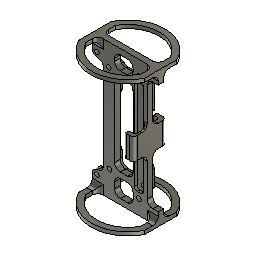
RISE_SensorMount (Autodesk Fusion 360 design; units mm, degrees)
Autodesk Fusion 360 part; units mm, degrees
(part 1 of 2)
sketch "Sketch1" plane through (0, 0, 0) normal (0, 0, 1) x (1, 0, 0)
  circle A0 centre (0, 0) radius 20
  line L0 (15, -5) -> (-15, -5)
  line L1 (-15, -5) -> (-15, 5)
  line L2 (-15, 5) -> (15, 5)
  line L3 (15, 5) -> (15, -5)
  line L4 (15, -5) -> (-15, 5) construction
  line L5 (-15, -5) -> (15, 5) construction
  dimension "d1" = 40
  dimension "d2" = 30
  dimension "d3" = 10
  constraint coincident A0.centre origin
  constraint horizontal L0
  constraint perpendicular L0 L1
  constraint parallel L0 L2
  constraint parallel L1 L3
  constraint coincident L4 A0.centre
  constraint coincident L5 A0.centre
  measures "d1" diameter of A0
  measures "d2" distance of L1.end L2.end
  measures "d3" distance of L0.end L1.end
extrude "Extrude1" add sketch "Sketch1" along normal blind 70 contours L0 L1 L2 L3 makes body 1
extrude "Extrude2" add sketch "Sketch1" against normal blind 3 separate body makes body 2
extrude "Extrude3" add sketch "Sketch1" against normal blind 3 contours L0 L1 L2 L3 bodies 1 2
sketch "Sketch2" plane through (0, 0, 70) normal (0, 0, 1) x (-1, 0, 0)
  line L0 (-15, -5) -> (15, -5)
  line L1 (15, -5) -> (15, 5)
  line L2 (15, 5) -> (-15, 5)
  line L3 (-15, 5) -> (-15, -5)
  circle A0 centre (0, 0) radius 20
  constraint coincident A0.centre origin
extrude "Extrude4" add sketch "Sketch2" along normal blind 3 contours L0 L1 L2 L3 | A0 bodies 1
sketch "Sketch3" plane through (0, -5, 0) normal (0, -1, 0) x (1, 0, 0)
  line L0 (-15, 0) -> (15, 0)
  line L1 (15, 0) -> (15, 70)
  line L2 (15, 70) -> (-15, 70)
  line L3 (-15, 70) -> (-15, 0)
  circle A0 centre (-11.5, 64) radius 1.25
  circle A1 centre (11.5, 64) radius 1.25
  circle A2 centre (-11.5, 6) radius 1.25
  circle A3 centre (11.5, 6) radius 1.25
  line L4 (-14, 59.5) -> (-14, 10.5)
  line L5 (-9, 10.5) -> (-9, 59.5)
  line L6 (9, 10.5) -> (9, 59.5)
  line L7 (14, 59.5) -> (14, 10.5)
  line L8 (10.5, 9) -> (12.5, 9)
  line L9 (10.5, 61) -> (12.5, 61)
  line L10 (-12.5, 61) -> (-10.5, 61)
  line L11 (-12.5, 9) -> (-10.5, 9)
  arc A4 (-12.5, 61) -> (-14, 59.5) centre (-12.5, 59.5) ccw
  arc A5 (-9, 59.5) -> (-10.5, 61) centre (-10.5, 59.5) ccw
  arc A6 (-14, 10.5) -> (-12.5, 9) centre (-12.5, 10.5) ccw
  arc A7 (-10.5, 9) -> (-9, 10.5) centre (-10.5, 10.5) ccw
  arc A8 (9, 10.5) -> (10.5, 9) centre (10.5, 10.5) ccw
  arc A9 (12.5, 9) -> (14, 10.5) centre (12.5, 10.5) ccw
  arc A10 (14, 59.5) -> (12.5, 61) centre (12.5, 59.5) ccw
  arc A11 (10.5, 61) -> (9, 59.5) centre (10.5, 59.5) ccw
  dimension "d13" = 23
  dimension "d14" = 58
  dimension "d15" = 2.5
  dimension "d16" = 2.5
  dimension "d17" = 2.5
  dimension "d18" = 2.5
  dimension "d20" = 1.5
  dimension "d21" = 1.5
  dimension "d22" = 1.5
  dimension "d23" = 1.5
  dimension "d24" = 1.5
  dimension "d25" = 1.5
  dimension "d26" = 1.5
  dimension "d27" = 1.5
  constraint perpendicular L7 L8
  constraint perpendicular L7 L9
  constraint perpendicular L5 L10
  constraint perpendicular L5 L11
  constraint tangent L4 A4
  constraint tangent L10 A4
  constraint tangent L5 A5
  constraint tangent L10 A5
  constraint tangent L4 A6
  constraint tangent L11 A6
  constraint tangent L5 A7
  constraint tangent L11 A7
  constraint tangent L6 A8
  constraint tangent L8 A8
  constraint tangent L8 A9
  constraint tangent L7 A9
  constraint tangent L7 A10
  constraint tangent L9 A10
  constraint tangent L6 A11
  constraint tangent L9 A11
  measures "d13" distance of A0.centre A1.centre
  measures "d14" distance of A0.centre A2.centre
  measures "d15" diameter of A0
  measures "d16" diameter of A1
  measures "d17" diameter of A2
  measures "d18" diameter of A3
  measures "d20" radius of A4
  measures "d21" radius of A5
  measures "d22" radius of A6
  measures "d23" radius of A7
  measures "d24" radius of A8
  measures "d25" radius of A9
  measures "d26" radius of A10
  measures "d27" radius of A11
extrude "Extrude5" cut sketch "Sketch3" against normal blind 2 contours L4 L5 L10 L11 A4 A5 A6 A7 | L6 L7 L8 L9 A8 A9 A10 A11 bodies 1
extrude "Extrude6" cut 1 faces at (3, -5, 26.8333) along direction (0, 1, 0) blind 2.5 on bodies 1 bodies 1
extrude "Extrude7" cut 2 faces at (-10.6667, -3, 26.8333) (12.3333, -3, 43.1667) along direction (0, 1, 0) blind 2.5 on bodies 1 bodies 1
extrude "Extrude8" cut 1 faces at (-5, 5, 23.3333) along direction (0, -1, 0) blind 2.5 on bodies 1 bodies 1
extrude "Extrude9" cut sketch "Sketch3" against normal blind 100 contours A2 | A3 bodies 1
extrude "Extrude10" cut sketch "Sketch3" against normal blind 100 contours A0 | A1 bodies 1
sketch "Sketch4" plane through (0, 2.5, 0) normal (0, 1, 0) x (-1, 0, 0)
  circle A0 centre (11.5, 64) radius 1.25
  circle A1 centre (-11.5, 64) radius 1.25
  circle A2 centre (11.5, 6) radius 1.25
  circle A3 centre (-11.5, 6) radius 1.25
  line L0 (-15, 0) -> (15, 0)
  line L1 (15, 0) -> (15, 70)
  line L2 (15, 70) -> (-15, 70)
  line L3 (-15, 70) -> (-15, 0)
  line L4 (0, 0) -> (0, 9)
  line L5 (0, 9) -> (0, 12)
  line L6 (0, 12) -> (7.25, 12)
  line L7 (0, 12) -> (-7.25, 12)
  circle A4 centre (-8.5, 12) radius 1.25
  circle A5 centre (8.5, 12) radius 1.25
  line L8 (0, 12) -> (0, 21.5)
  line L9 (0, 0) -> (0, 21.5)
  line L10 (0, 24.5) -> (0, 35)
  line L11 (0, 70) -> (0, 60)
  line L12 (0, 60) -> (9, 60)
  line L13 (0, 60) -> (-9, 60)
  line L14 (0, 60) -> (0, 45)
  line L15 (9.5, 43.5) -> (-9.5, 43.5)
  line L16 (-10.5, 44.5) -> (-10.5, 45.5)
  line L17 (-9.5, 46.5) -> (9.5, 46.5)
  line L18 (10.5, 45.5) -> (10.5, 44.5)
  line L19 (10.5, 43.5) -> (-10.5, 46.5) construction
  line L20 (-10.5, 43.5) -> (10.5, 46.5) construction
  line L21 (0, 35) -> (0, 45)
  line L22 (0, 21.5) -> (0, 23)
  line L23 (8.5, 24.5) -> (-8.5, 24.5)
  line L24 (-9.5, 23.5) -> (-9.5, 22.5)
  line L25 (-8.5, 21.5) -> (8.5, 21.5)
  line L26 (9.5, 22.5) -> (9.5, 23.5)
  line L27 (9.5, 24.5) -> (-9.5, 21.5) construction
  line L28 (-9.5, 24.5) -> (9.5, 21.5) construction
  circle A6 centre (-9, 60) radius 1.25
  circle A7 centre (9, 60) radius 1.25
  arc A8 (-9.5, 46.5) -> (-10.5, 45.5) centre (-9.5, 45.5) ccw
  arc A9 (-10.5, 44.5) -> (-9.5, 43.5) centre (-9.5, 44.5) ccw
  arc A10 (10.5, 45.5) -> (9.5, 46.5) centre (9.5, 45.5) ccw
  arc A11 (9.5, 43.5) -> (10.5, 44.5) centre (9.5, 44.5) ccw
  arc A12 (-9.5, 22.5) -> (-8.5, 21.5) centre (-8.5, 22.5) ccw
  arc A13 (-8.5, 24.5) -> (-9.5, 23.5) centre (-8.5, 23.5) ccw
  arc A14 (9.5, 23.5) -> (8.5, 24.5) centre (8.5, 23.5) ccw
  arc A15 (8.5, 21.5) -> (9.5, 22.5) centre (8.5, 22.5) ccw
  point P0 (0, 45)
  point P1 (0, 23)
  dimension "d40" = 9
  dimension "d48" = 3
  dimension "d49" = 8.5
  dimension "d50" = 8.5
  dimension "d51" = 2.5
  dimension "d52" = 2.5
  dimension "d74" = 35
  dimension "d75" = 10
  dimension "d76" = 9
  dimension "d77" = 9
  dimension "d78" = 15
  dimension "d79" = 21
  dimension "d80" = 3
  dimension "d81" = 19
  dimension "d82" = 3
  dimension "d83" = 2.5
  dimension "d84" = 2.5
  dimension "d85" = 1
  dimension "d86" = 1
  dimension "d87" = 1
  dimension "d88" = 1
  dimension "d89" = 1
  dimension "d90" = 1
  dimension "d91" = 1
  dimension "d92" = 1
  constraint coincident L4.start L9.start
  constraint perpendicular L0 L4
  constraint parallel L4 L5
  constraint perpendicular L5 L6
  constraint perpendicular L5 L7
  constraint coincident A5 L6.end
  constraint coincident A4 L7.end
  constraint collinear L9 L10
  constraint midpoint L2 L11.start
  constraint perpendicular L2 L11
  constraint perpendicular L11 L12
  constraint perpendicular L11 L13
  constraint perpendicular L12 L14
  constraint horizontal L15
  constraint perpendicular L15 L16
  constraint parallel L15 L17
  constraint parallel L16 L18
  constraint coincident L19 P0
  constraint coincident L20 P0
  constraint coincident P0 L14.end
  constraint parallel L8 L22
  constraint horizontal L23
  constraint perpendicular L23 L24
  constraint parallel L23 L25
  constraint parallel L24 L26
  constraint coincident L27 P1
  constraint coincident L28 P1
  constraint coincident P1 L22.end
  constraint coincident L13.end A6.centre
  constraint coincident L12.end A7.centre
  constraint coincident L19.end L16
  constraint coincident L19.end L17
  constraint tangent L16 A8
  constraint tangent L17 A8
  constraint coincident L20.start L16
  constraint coincident L20.start L15
  constraint tangent L16 A9
  constraint tangent L15 A9
  constraint coincident L20.end L17
  constraint coincident L20.end L18
  constraint tangent L17 A10
  constraint tangent L18 A10
  constraint coincident L19.start L15
  constraint coincident L19.start L18
  constraint tangent L15 A11
  constraint tangent L18 A11
  constraint coincident L27.end L25
  constraint coincident L27.end L24
  constraint tangent L25 A12
  constraint tangent L24 A12
  constraint coincident L28.start L24
  constraint coincident L28.start L23
  constraint tangent L24 A13
  constraint tangent L23 A13
  constraint coincident L27.start L23
  constraint coincident L27.start L26
  constraint tangent L23 A14
  constraint tangent L26 A14
  constraint coincident L28.end L25
  constraint coincident L28.end L26
  constraint tangent L25 A15
  constraint tangent L26 A15
  measures "d40" distance of L4.start L4.end
  measures "d48" distance of L4.end L5.end
  measures "d49" distance of L5.end A5.centre
  measures "d50" distance of L5.end A4.centre
  measures "d51" diameter of A4
  measures "d52" diameter of A5
  measures "d74" distance of L4.start L10.end
  measures "d75" distance of L11.start L11.end
  measures "d76" distance of L11.end L12.end
  measures "d77" distance of L11.end L13.end
  measures "d78" distance of L11.end P0
  measures "d79" distance of L19.end L20.end
  measures "d80" distance of L20.start L19.end
  measures "d81" distance of L27.end L28.end
  measures "d82" distance of L28.start L27.end
  measures "d83" diameter of A6
  measures "d84" diameter of A7
  measures "d85" radius of A8
  measures "d86" radius of A9
  measures "d87" radius of A10
  measures "d88" radius of A11
  measures "d89" radius of A12
  measures "d90" radius of A13
  measures "d91" radius of A14
  measures "d92" radius of A15
extrude "Extrude15" cut sketch "Sketch4" against normal blind 100 contours A6 bodies 1
extrude "Extrude16" cut sketch "Sketch4" against normal blind 100 contours A4 | A5 | A7 bodies 1
extrude "Extrude17" cut sketch "Sketch4" against normal blind 2 contours L23 L24 L25 L26 A12 A13 A14 A15 | L14 L15 L17 L18 L21 A10 A11 | L14 L15 L16 L17 L21 A8 A9 bodies 1
extrude "Extrude18" add 1 faces at (-15, -0.8333, 23.3333) along direction (-1, 0, 0) blind 3 on bodies 1 bodies 1
extrude "Extrude19" add 1 faces at (15, 0.8333, 23.3333) along direction (1, 0, 0) blind 3 on bodies 1 bodies 1
sketch "Sketch5" plane through (0, 0, 70) normal (0, 0, -1) x (1, 0, 0)
  line L0 (18, -2.5) -> (-18, -2.5)
  line L1 (-18, -2.5) -> (-18, 2.5)
  line L2 (-18, 2.5) -> (18, 2.5)
  line L3 (18, 2.5) -> (18, -2.5)
  circle A0 centre (0, 0) radius 20
  line L4 (18, -2.5) -> (18, -8.7178)
  line L5 (18, -8.7178) -> (18, 2.5)
  line L6 (18, 2.5) -> (18, 8.7178)
  line L7 (-18, 2.5) -> (-18, 8.7178)
  line L8 (-18, -2.5) -> (-18, -8.7178)
  constraint coincident L0.start L3.end
  constraint coincident A0 L4.end
  constraint perpendicular L0 L4
  constraint coincident L2.end L3.start
  constraint coincident A0 L6.end
  constraint perpendicular L2 L6
  constraint coincident L1.end L2.start
  constraint coincident A0 L7.end
  constraint perpendicular L2 L7
  constraint coincident L0.end L1.start
  constraint coincident A0 L8.end
  constraint perpendicular L0 L8
extrude "Extrude20" cut sketch "Sketch5" against normal blind 10 contours L3 A0 L4 L5 L6 | L1 A0 L7 L8 bodies 1
sketch "Sketch6" plane through (0, 0, 0) normal (0, 0, 1) x (-1, 0, 0)
  line L0 (-18, 2.5) -> (18, 2.5)
  line L1 (18, 2.5) -> (18, -2.5)
  line L2 (18, -2.5) -> (-18, -2.5)
  line L3 (-18, -2.5) -> (-18, 2.5)
  circle A0 centre (0, 0) radius 20
  line L4 (18, 2.5) -> (18, 8.7178)
  line L5 (18, 8.7178) -> (18, -8.7178)
  line L6 (-18, -2.5) -> (-18, -8.7178)
  line L7 (-18, -8.7178) -> (-18, 8.7178)
  constraint coincident L0.end L1.start
  constraint coincident A0 L4.end
  constraint perpendicular L0 L4
  constraint coincident A0 L5.end
  constraint perpendicular L2 L5
  constraint coincident L2.end L3.start
  constraint coincident A0 L6.end
  constraint perpendicular L2 L6
  constraint coincident A0 L7.end
  constraint perpendicular L0 L7
extrude "Extrude21" cut sketch "Sketch6" against normal blind 10 contours L3 A0 L6 L7 bodies 1
extrude "Extrude22" cut sketch "Sketch6" against normal blind 10 contours L1 A0 L4 L5 bodies 1
extrude "Extrude23" cut 2 faces at (-12.3867, -0.5, 27.6871) (12.3867, -0.5, 27.6871) along direction (0, 1, 0) blind 1 on bodies 1 bodies 1
extrude "Extrude24" cut 1 faces at (-2.7544, -2.5, 43.6171) along direction (0, 1, 0) blind 1 on bodies 1 bodies 1
extrude "Extrude25" cut 1 faces at (-2.8333, 2.5, 37.1667) along direction (0, -1, 0) blind 1 on bodies 1 bodies 1
extrude "Extrude26" cut 2 faces at (3, 0.5, 44.5) (-2.8333, 0.5, 22.5) along direction (0, -1, 0) blind 1 on bodies 1 bodies 1
extrude "Extrude27" cut 1 faces at (6.499, 3.7661, 73) along direction (0, 0, -1) blind 1 on bodies 1 bodies 1
extrude "Extrude28" cut 1 faces at (4.8796, -1.2694, -3) along direction (0, 0, 1) blind 1 on bodies 1 bodies 1
sketch "Sketch7" plane through (0, 0, -2) normal (0, 0, -1) x (1, 0, 0)
  line L0 (-18, 8.7178) -> (-18, -8.7178)
  arc A0 (-18, -8.7178) -> (18, -8.7178) centre (0, 0) ccw
  line L1 (18, -8.7178) -> (18, 8.7178)
  arc A1 (18, 8.7178) -> (-18, 8.7178) centre (0, 0) ccw
  circle A2 centre (0, 0) radius 17
  line L2 (-18, 0) -> (-15, 0)
  line L3 (-15, 0) -> (-15, 8)
  line L4 (-15, 0) -> (-15, -8)
  line L5 (18, 0) -> (15, 0)
  line L6 (15, 0) -> (15, -8)
  line L7 (15, 0) -> (15, 8)
  line L8 (0, 0) -> (0, 1.5)
  line L9 (0, 0) -> (0, -1.5)
  line L10 (0, -1.5) -> (15, -1.5)
  line L11 (0, -1.5) -> (-15, -1.5)
  line L12 (0, 1.5) -> (-15, 1.5)
  line L13 (0, 1.5) -> (15, 1.5)
  dimension "d131" = 34
  dimension "d132" = 1.5
  dimension "d133" = 1.5
  constraint concentric A0 A2
  constraint midpoint L0 L2.start
  constraint perpendicular L0 L2
  constraint coincident A2 L3.end
  constraint perpendicular L2 L3
  constraint coincident A2 L4.end
  constraint perpendicular L2 L4
  constraint midpoint L1 L5.start
  constraint perpendicular L1 L5
  constraint coincident A2 L6.end
  constraint perpendicular L5 L6
  constraint coincident A2 L7.end
  constraint perpendicular L5 L7
  constraint coincident A0.centre A1.centre
  constraint parallel L6 L8
  constraint parallel L8 L9
  constraint coincident L6 L10.end
  constraint perpendicular L6 L10
  constraint coincident L4 L11.end
  constraint perpendicular L4 L11
  constraint perpendicular L8 L12
  constraint coincident L7 L13.end
  constraint perpendicular L7 L13
  measures "d131" diameter of A2
  measures "d132" distance of A0.centre L8.end
  measures "d133" distance of A0.centre L9.end
extrude "Extrude29" cut sketch "Sketch7" against normal blind 100 contours A2 L3 L7 L12 L13 | A2 L4 L6 L10 L11 bodies 1
sketch "Sketch8" plane through (0, -1.5, 0) normal (0, -1, 0) x (1, 0, 0)
  arc A0 (-9, 58.75) -> (-9.895, 60.8726) centre (-9, 60) ccw
  line L0 (-9, 58.75) -> (-9, 13.1456)
  arc A1 (-9, 10.8544) -> (-9, 13.1456) centre (-8.5, 12) ccw
  line L1 (-9, 10.8544) -> (-9, 10.5)
  arc A2 (-10.5, 9) -> (-9, 10.5) centre (-10.5, 10.5) ccw
  line L2 (-10.5, 9) -> (-12.5, 9)
  arc A3 (-14, 10.5) -> (-12.5, 9) centre (-12.5, 10.5) ccw
  line L3 (-14, 10.5) -> (-14, 59.5)
  arc A4 (-12.5, 61) -> (-14, 59.5) centre (-12.5, 59.5) ccw
  line L4 (-12.5, 61) -> (-10.5, 61)
  arc A5 (-9.895, 60.8726) -> (-10.5, 61) centre (-10.5, 59.5) ccw
  arc A6 (9, 13.1456) -> (9, 10.8544) centre (8.5, 12) ccw
  line L5 (9, 13.1456) -> (9, 58.75)
  arc A7 (9.895, 60.8726) -> (9, 58.75) centre (9, 60) ccw
  arc A8 (10.5, 61) -> (9.895, 60.8726) centre (10.5, 59.5) ccw
  line L6 (10.5, 61) -> (12.5, 61)
  arc A9 (14, 59.5) -> (12.5, 61) centre (12.5, 59.5) ccw
  line L7 (14, 59.5) -> (14, 10.5)
  arc A10 (12.5, 9) -> (14, 10.5) centre (12.5, 10.5) ccw
  line L8 (12.5, 9) -> (10.5, 9)
  arc A11 (9, 10.5) -> (10.5, 9) centre (10.5, 10.5) ccw
  line L9 (9, 10.5) -> (9, 10.8544)
  circle A12 centre (11.5, 6) radius 1.25
  circle A13 centre (-11.5, 6) radius 1.25
  circle A14 centre (11.5, 64) radius 1.25
  circle A15 centre (-11.5, 64) radius 1.25
  line L10 (15, 70) -> (15, 72)
  line L11 (15, 72) -> (-15, 72)
  line L12 (-15, 72) -> (-15, 70)
  line L13 (-18, 70) -> (-18, 0)
  line L14 (-15, 0) -> (-15, -2)
  line L15 (-15, -2) -> (15, -2)
  line L16 (15, -2) -> (15, 0)
  line L17 (18, 0) -> (18, 70)
  line L18 (0, -2) -> (-6, -2)
  line L19 (0, -2) -> (6, -2)
  line L20 (6, 7) -> (6, 63)
  line L21 (6, 72) -> (-6, 72)
  line L22 (-6, 63) -> (-6, 7)
  line L23 (6, -2) -> (6, 35)
  line L24 (6, 35) -> (0, 35)
  line L25 (6, -2) -> (6, 4)
  line L26 (-6, -2) -> (-6, 4)
  line L27 (6, 72) -> (6, 66)
  line L28 (3, 66) -> (-3, 66)
  line L29 (3, 4) -> (-3, 4)
  arc A16 (6, 63) -> (3, 66) centre (3, 63) ccw
  arc A17 (-3, 66) -> (-6, 63) centre (-3, 63) ccw
  arc A18 (3, 4) -> (6, 7) centre (3, 7) ccw
  arc A19 (-6, 7) -> (-3, 4) centre (-3, 7) ccw
  line L30 (15, 0) -> (18, 0)
  line L31 (18, 70) -> (15, 70)
  line L32 (-15, 70) -> (-18, 70)
  line L33 (-18, 0) -> (-15, 0)
  dimension "d138" = 6
  dimension "d139" = 6
  dimension "d140" = 12
  dimension "d141" = 6
  dimension "d142" = 6
  dimension "d143" = 6
  dimension "d144" = 3
  dimension "d145" = 3
  dimension "d146" = 3
  dimension "d147" = 3
  constraint midpoint L15 L18.start
  constraint perpendicular L0 L18
  constraint perpendicular L5 L19
  constraint coincident L11 L21.start
  constraint perpendicular L11 L20
  constraint perpendicular L20 L21
  constraint perpendicular L20 L24
  constraint perpendicular L15 L25
  constraint perpendicular L15 L26
  constraint perpendicular L11 L27
  constraint perpendicular L22 L28
  constraint coincident L20 L23.end
  constraint coincident L21.start L20
  constraint coincident L27.end L28
  constraint tangent L20 A16
  constraint tangent L28 A16
  constraint coincident L21.end L22
  constraint tangent L28 A17
  constraint tangent L22 A17
  constraint coincident L19.end L20
  constraint coincident L25.end L29
  constraint tangent L20 A18
  constraint tangent L29 A18
  constraint coincident L26.end L29
  constraint coincident L18.end L22
  constraint tangent L29 A19
  constraint tangent L22 A19
  measures "d138" distance of L18.start L18.end
  measures "d139" distance of L18.start L19.end
  measures "d140" distance of L21.start L21.end
  measures "d141" distance of L19.end L25.end
  measures "d142" distance of L18.end L26.end
  measures "d143" distance of L21.start L27.end
  measures "d144" radius of A16
  measures "d145" radius of A17
  measures "d146" radius of A18
  measures "d147" radius of A19
move_body "Move1" bodies 1 to x (1, 0, 0) y (0, 1, 0) z (0, 0, 1) at (3, 0, 0)
extrude "Extrude31" add 2 faces at (-8.1449, 0.5, 54.9242) (14.1491, 0.5, 54.9261) along direction (0, -1, 0) blind 2 on bodies 1 bodies 1
sketch "Sketch9" plane through (0, -1.5, 0) normal (0, -1, 0) x (1, 0, 0)
  circle A0 centre (12, 60) radius 1.25
  line L0 (12, 46.5) -> (12.5, 46.5)
  arc A1 (13.5, 45.5) -> (12.5, 46.5) centre (12.5, 45.5) ccw
  line L1 (13.5, 45.5) -> (13.5, 44.5)
  arc A2 (12.5, 43.5) -> (13.5, 44.5) centre (12.5, 44.5) ccw
  line L2 (12.5, 43.5) -> (12, 43.5)
  line L3 (12, 43.5) -> (12, 46.5)
  circle A3 centre (11.5, 12) radius 1.25
  circle A4 centre (-5.5, 12) radius 1.25
  arc A5 (-6.5, 22.5) -> (-6, 21.634) centre (-5.5, 22.5) ccw
  line L4 (-6.5, 22.5) -> (-6.5, 23.5)
  arc A6 (-6, 24.366) -> (-6.5, 23.5) centre (-5.5, 23.5) ccw
  line L5 (-6, 24.366) -> (-6, 21.634)
  circle A7 centre (-6, 60) radius 1.25
  line L6 (-6, 43.5) -> (-6.5, 43.5)
  arc A8 (-7.5, 44.5) -> (-6.5, 43.5) centre (-6.5, 44.5) ccw
  line L7 (-7.5, 44.5) -> (-7.5, 45.5)
  arc A9 (-6.5, 46.5) -> (-7.5, 45.5) centre (-6.5, 45.5) ccw
  line L8 (-6.5, 46.5) -> (-6, 46.5)
  line L9 (-6, 46.5) -> (-6, 43.5)
  arc A10 (12.5, 23.5) -> (12, 24.366) centre (11.5, 23.5) ccw
  line L10 (12.5, 23.5) -> (12.5, 22.5)
  arc A11 (12, 21.634) -> (12.5, 22.5) centre (11.5, 22.5) ccw
  line L11 (12, 21.634) -> (12, 24.366)
  circle A12 centre (14.5, 6) radius 1.25
  circle A13 centre (-8.5, 6) radius 1.25
  circle A14 centre (14.5, 64) radius 1.25
  circle A15 centre (-8.5, 64) radius 1.25
  line L12 (18, 70) -> (18, 72)
  line L13 (18, 72) -> (-12, 72)
  line L14 (-12, 72) -> (-12, 70)
  line L15 (-15, 70) -> (-15, 0)
  line L16 (-12, 0) -> (-12, -2)
  line L17 (-12, -2) -> (18, -2)
  line L18 (18, -2) -> (18, 0)
  line L19 (21, 0) -> (21, 70)
  line L20 (-10, 66) -> (16, 66)
  line L21 (16, 66) -> (16, 4)
  line L22 (16, 4) -> (-10, 4)
  line L23 (-10, 4) -> (-10, 66)
  line L24 (18, 0) -> (21, 0)
  line L25 (21, 70) -> (18, 70)
  line L26 (-12, 70) -> (-15, 70)
  line L27 (-15, 0) -> (-12, 0)
  constraint horizontal L20
  constraint vertical L21
  constraint horizontal L22
  constraint vertical L23
extrude "Extrude32" add sketch "Sketch9" against normal blind 1 contours L0 A1 L1 A2 L2 L3 | A5 L4 A6 L5 | L6 A8 L7 A9 L8 L9 | A10 L10 A11 L11 bodies 1
extrude "Extrude33" add sketch "Sketch9" against normal blind 3 contours A12 | A13 | A14 | A15 bodies 1
extrude "Extrude34" cut sketch "Sketch3" against normal blind 5 contours L4 L5 L10 L11 A4 A5 A6 A7 | L6 L7 L8 L9 A8 A9 A10 A11 bodies 1
move_body "Move2" bodies 1 to x (1, 0, 0) y (0, 1, 0) z (0, 0, 1) at (1, 0, 0)
extrude "Extrude35" cut sketch "Sketch3" against normal blind 100 contours A0 | A1 | A2 | A3 bodies 1
extrude "Extrude36" add 1 faces at (12, 0, 37.1667) along direction (0, -1, 0) blind 1.5 on bodies 1 bodies 1
extrude "Extrude37" cut sketch "Sketch3" against normal blind 5 contours L6 L7 L8 L9 A8 A9 A10 A11 bodies 1
extrude "Extrude38" add 1 faces at (-9.6667, 0, 26.8333) along direction (0, -1, 0) blind 2 on bodies 1 bodies 1
extrude "Extrude39" cut 1 faces at (-9.6667, -2, 26.8333) along direction (0, 1, 0) blind 0.5 on bodies 1 bodies 1
extrude "Extrude40" add 2 faces at (11.7309, 0, 50.5961) (11.6667, 0, 37.1667) along direction (0, -1, 0) blind 0.5 on bodies 1 bodies 1
sketch "Sketch10" plane through (22, 0, 0) normal (1, 0, 0) x (0, 1, 0)
  line L0 (-8.7178, -2) -> (8.7178, -2)
  line L1 (8.7178, -2) -> (8.7178, 0)
  line L2 (8.7178, 0) -> (1.5, 0)
  line L3 (1.5, 0) -> (1.5, 70)
  line L4 (1.5, 70) -> (8.7178, 70)
  line L5 (8.7178, 70) -> (8.7178, 72)
  line L6 (8.7178, 72) -> (-8.7178, 72)
  line L7 (-8.7178, 72) -> (-8.7178, 70)
  line L8 (-8.7178, 70) -> (-1.5, 70)
  line L9 (-1.5, 70) -> (-1.5, 0)
  line L10 (-1.5, 0) -> (-8.7178, 0)
  line L11 (-8.7178, 0) -> (-8.7178, -2)
  line L12 (0, -2) -> (0, 5)
  line L13 (0, 72) -> (0, 65)
  line L14 (0, 5) -> (0, 65)
  line L15 (1.5, 65) -> (-1.5, 65)
  line L16 (-1.5, 65) -> (-1.5, 5)
  line L17 (-1.5, 5) -> (1.5, 5)
  line L18 (1.5, 5) -> (1.5, 65)
  line L19 (1.5, 65) -> (-1.5, 5) construction
  line L20 (-1.5, 65) -> (1.5, 5) construction
  point P0 (0, 35)
  dimension "d170" = 7
  dimension "d171" = 7
  dimension "d172" = 60
  constraint midpoint L0 L12.start
  constraint perpendicular L6 L12
  constraint midpoint L6 L13.start
  constraint perpendicular L6 L13
  constraint horizontal L15
  constraint perpendicular L15 L16
  constraint parallel L15 L17
  constraint parallel L16 L18
  constraint coincident L19 P0
  constraint coincident L20 P0
  constraint midpoint L14 P0
  measures "d170" distance of L12.start L12.end
  measures "d171" distance of L13.start L13.end
  measures "d172" distance of L15.end L16.end
extrude "Extrude41" cut sketch "Sketch10" against normal blind 7 contours L9 L14 L15 L16 L17 | L3 L14 L15 L17 L18 bodies 1
sketch "Sketch11" plane through (0, -1.5, 0) normal (0, -1, 0) x (1, 0, 0)
  line L0 (15, 65) -> (22, 65)
  line L1 (22, 65) -> (22, 70)
  line L2 (22, 70) -> (19, 70)
  line L3 (19, 70) -> (19, 72)
  line L4 (19, 72) -> (-11, 72)
  line L5 (-11, 72) -> (-11, 70)
  line L6 (-11, 70) -> (-14, 70)
  line L7 (-14, 70) -> (-14, 0)
  line L8 (-14, 0) -> (-11, 0)
  line L9 (-11, 0) -> (-11, -2)
  line L10 (-11, -2) -> (19, -2)
  line L11 (19, -2) -> (19, 0)
  line L12 (19, 0) -> (22, 0)
  line L13 (22, 0) -> (22, 5)
  line L14 (22, 5) -> (15, 5)
  line L15 (15, 5) -> (15, 65)
  line L16 (10.5, 61) -> (12.25, 61)
  arc A0 (14, 59.25) -> (12.25, 61) centre (13, 60) ccw
  line L17 (14, 59.25) -> (14, 46.366)
  arc A1 (14.5, 45.5) -> (14, 46.366) centre (13.5, 45.5) ccw
  line L18 (14.5, 45.5) -> (14.5, 44.5)
  arc A2 (14, 43.634) -> (14.5, 44.5) centre (13.5, 44.5) ccw
  line L19 (14, 43.634) -> (14, 10.5)
  arc A3 (12.5, 9) -> (14, 10.5) centre (12.5, 10.5) ccw
  line L20 (12.5, 9) -> (10.5, 9)
  arc A4 (9, 10.5) -> (10.5, 9) centre (10.5, 10.5) ccw
  arc A5 (10.5, 61) -> (9, 59.5) centre (10.5, 59.5) ccw
  circle A6 centre (-11.5, 6) radius 1.25
  circle A7 centre (11.5, 6) radius 1.25
  circle A8 centre (-11.5, 64) radius 1.25
  circle A9 centre (11.5, 64) radius 1.25
  circle A10 centre (-5, 60) radius 1.25
  circle A11 centre (-4.5, 12) radius 1.25
  line L21 (14, 43.634) -> (14, 46.366)
  line L22 (9, 10.5) -> (9, 59.5)
  constraint coincident A2.start L19.start
  constraint coincident L17.end A1.end
extrude "Extrude42" add sketch "Sketch11" against normal blind 3 contours A1 L18 A2 L21 bodies 1
sketch "Sketch13" plane through (15, 0, 0) normal (1, 0, 0) x (0, 1, 0)
  line L0 (-1.5, 65) -> (-1.5, 5)
  line L1 (1.5, 5) -> (1.5, 65)
  line L2 (0, 7) -> (0, 63)
  line L3 (9, 41) -> (-9, 41)
  line L4 (-9, 41) -> (-9, 29)
  line L5 (-9, 29) -> (9, 29)
  line L6 (9, 29) -> (9, 41)
  line L7 (9, 41) -> (-9, 29) construction
  line L8 (-9, 41) -> (9, 29) construction
  line L9 (1.5, 65) -> (-1.5, 65)
  line L10 (-1.5, 5) -> (1.5, 5)
  point P0 (0, 35)
  dimension "d192" = 18
  dimension "d193" = 12
  constraint horizontal L3
  constraint perpendicular L3 L4
  constraint parallel L3 L5
  constraint parallel L4 L6
  constraint coincident L7 P0
  constraint coincident L8 P0
  constraint midpoint L2 P0
  measures "d192" distance of L4.end L5.end
  measures "d193" distance of L3.end L4.end
extrude "Extrude45" add sketch "Sketch13" along normal blind 1 contours L0 L2 L3 L5 | L0 L3 L4 L5 | L1 L2 L3 L5 | L1 L3 L5 L6 bodies 1
sketch "Sketch14" plane through (-14, 0, 0) normal (-1, 0, 0) x (0, -1, 0)
  line L0 (-8.7178, -2) -> (8.7178, -2)
  line L1 (8.7178, -2) -> (8.7178, 0)
  line L2 (8.7178, 0) -> (1.5, 0)
  line L3 (1.5, 0) -> (1.5, 70)
  line L4 (1.5, 70) -> (8.7178, 70)
  line L5 (8.7178, 70) -> (8.7178, 72)
  line L6 (8.7178, 72) -> (-8.7178, 72)
  line L7 (-8.7178, 72) -> (-8.7178, 70)
  line L8 (-8.7178, 70) -> (-1.5, 70)
  line L9 (-1.5, 70) -> (-1.5, 0)
  line L10 (-1.5, 0) -> (-8.7178, 0)
  line L11 (-8.7178, 0) -> (-8.7178, -2)
  line L12 (0, -2) -> (0, 72)
  line L13 (1.5, 60) -> (-1.5, 60)
  line L14 (-1.5, 60) -> (-1.5, 10)
  line L15 (-1.5, 10) -> (1.5, 10)
  line L16 (1.5, 10) -> (1.5, 60)
  line L17 (1.5, 60) -> (-1.5, 10) construction
  line L18 (-1.5, 60) -> (1.5, 10) construction
  point P0 (0, 35)
  dimension "d196" = 50
  constraint midpoint L0 L12.start
  constraint midpoint L6 L12.end
  constraint horizontal L13
  constraint perpendicular L13 L14
  constraint parallel L13 L15
  constraint parallel L14 L16
  constraint coincident L17 P0
  constraint coincident L18 P0
  constraint midpoint L12 P0
  measures "d196" distance of L13.end L14.end
extrude "Extrude46" cut sketch "Sketch14" against normal blind 5 contours L9 L12 L13 L14 L15 | L3 L12 L13 L15 L16 bodies 1
extrude "Extrude47" cut 1 faces at (-9, -0.5, 26.6667) along direction (1, 0, 0) blind 1 on bodies 1 bodies 1
extrude "Extrude48" cut 1 faces at (-12, 0.5, 10) along direction (0, 0, -1) blind 1.5 on bodies 1 bodies 1
extrude "Extrude49" cut 1 faces at (-10, 0.5, 60) along direction (0, 0, 1) blind 1.5 on bodies 1 bodies 1
extrude "Extrude50" add 2 faces at (15, -0.5, 13) (15, -0.5, 57) along direction (1, 0, 0) blind 1 on bodies 1 bodies 1
extrude "Extrude52" add 2 faces at (4.1667, -0.5, 44.5) (4.5, -0.5, 22.5) along direction (0, 1, 0) blind 0.5 on bodies 1 bodies 1
sketch "Sketch15" plane through (9, 0, 0) normal (1, 0, 0) x (0, 1, 0)
  line L0 (-0.5, 24.5) -> (-0.5, 43.5)
  line L1 (-0.5, 43.5) -> (0, 43.5)
  line L2 (0, 43.5) -> (0, 46.5)
  line L3 (0, 46.5) -> (-0.5, 46.5)
  line L4 (-0.5, 46.5) -> (-0.5, 59.5)
  line L5 (-0.5, 59.5) -> (-1.5, 59.5)
  line L6 (-1.5, 59.5) -> (-1.5, 10.5)
  line L7 (-1.5, 10.5) -> (-0.5, 10.5)
  line L8 (-0.5, 10.5) -> (-0.5, 21.5)
  line L9 (-0.5, 21.5) -> (0, 21.5)
  line L10 (0, 21.5) -> (0, 24.5)
  line L11 (0, 24.5) -> (-0.5, 24.5)
  line L12 (-0.5, 21.5) -> (-0.5, 24.5)
  line L13 (-0.5, 46.5) -> (-0.5, 43.5)
  constraint coincident L8.end L9.start
  constraint coincident L0.start L11.end
  constraint coincident L3.end L4.start
  constraint coincident L0.end L1.start
extrude "Extrude53" add sketch "Sketch15" along normal blind 5 contours L1 L2 L3 L13 bodies 1
extrude "Extrude54" add sketch "Sketch15" along normal blind 5 contours L9 L10 L11 L12 bodies 1
sketch "Sketch16" plane through (0, 1.5, 0) normal (0, 1, 0) x (-1, 0, 0)
  line L0 (-15, 29) -> (-16, 29)
  line L1 (-16, 29) -> (-16, 5)
  line L2 (-16, 5) -> (-22, 5)
  line L3 (-22, 5) -> (-22, 0)
  line L4 (-22, 0) -> (-19, 0)
  line L5 (-19, 0) -> (-19, -2)
  line L6 (-19, -2) -> (11, -2)
  line L7 (11, -2) -> (11, 0)
  line L8 (11, 0) -> (14, 0)
  line L9 (14, 0) -> (14, 8.5)
  line L10 (14, 8.5) -> (8, 8.5)
  line L11 (8, 8.5) -> (8, 61.5)
  line L12 (8, 61.5) -> (14, 61.5)
  line L13 (14, 61.5) -> (14, 70)
  line L14 (14, 70) -> (11, 70)
  line L15 (11, 70) -> (11, 72)
  line L16 (11, 72) -> (-19, 72)
  line L17 (-19, 72) -> (-19, 70)
  line L18 (-19, 70) -> (-22, 70)
  line L19 (-22, 70) -> (-22, 65)
  line L20 (-22, 65) -> (-16, 65)
  line L21 (-16, 65) -> (-16, 41)
  line L22 (-16, 41) -> (-15, 41)
  line L23 (5.5, 23.5) -> (5.5, 22.5)
  arc A0 (4.5, 21.5) -> (5.5, 22.5) centre (4.5, 22.5) ccw
  line L24 (4.5, 21.5) -> (-12.5, 21.5)
  arc A1 (-13.5, 22.5) -> (-12.5, 21.5) centre (-12.5, 22.5) ccw
  line L25 (-13.5, 22.5) -> (-13.5, 23.5)
  arc A2 (-12.5, 24.5) -> (-13.5, 23.5) centre (-12.5, 23.5) ccw
  line L26 (-12.5, 24.5) -> (4.5, 24.5)
  arc A3 (5.5, 23.5) -> (4.5, 24.5) centre (4.5, 23.5) ccw
  line L27 (5.5, 43.5) -> (-13.5, 43.5)
  arc A4 (-14, 43.634) -> (-13.5, 43.5) centre (-13.5, 44.5) ccw
  line L28 (-14, 43.634) -> (-14, 46.366)
  arc A5 (-13.5, 46.5) -> (-14, 46.366) centre (-13.5, 45.5) ccw
  line L29 (-13.5, 46.5) -> (5.5, 46.5)
  arc A6 (6.5, 45.5) -> (5.5, 46.5) centre (5.5, 45.5) ccw
  line L30 (6.5, 45.5) -> (6.5, 44.5)
  arc A7 (5.5, 43.5) -> (6.5, 44.5) centre (5.5, 44.5) ccw
  circle A8 centre (5, 60) radius 1.25
  circle A9 centre (4.5, 12) radius 1.25
  circle A10 centre (-12.5, 12) radius 1.25
  circle A11 centre (-13, 60) radius 1.25
  circle A12 centre (-11.5, 64) radius 1.25
  circle A13 centre (11.5, 64) radius 1.25
  circle A14 centre (-11.5, 6) radius 1.25
  circle A15 centre (11.5, 6) radius 1.25
  line L31 (6.5, 45) -> (-14.5, 45)
  line L32 (-14.5, 45) -> (-14.5, 43.5)
  line L33 (-14.5, 45) -> (-14.5, 46.5)
  line L34 (-14.5, 46.5) -> (-13, 46.5)
  line L35 (-14.5, 43.5) -> (-13, 43.5)
  line L36 (-13, 43.5) -> (-13, 46.5)
  line L37 (-15, 41) -> (-15, 29)
  dimension "d219" = 21
  dimension "d220" = 1.5
  dimension "d221" = 1.5
  constraint midpoint L30 L31.start
  constraint perpendicular L28 L31
  constraint perpendicular L31 L32
  constraint perpendicular L31 L33
  constraint coincident L29 L34.end
  constraint perpendicular L28 L34
  constraint coincident L27 L35.end
  constraint perpendicular L28 L35
  constraint perpendicular L31 L36
  measures "d219" distance of L31.start L31.end
  measures "d220" distance of L31.end L32.end
  measures "d221" distance of L31.end L33.end
extrude "Extrude55" cut sketch "Sketch16" against normal blind 1.5 contours A4 L28 L31 L32 L35 | L28 A5 L31 L33 L34 bodies 1
fillet "Fillet12" radius 1 2 edges at (14.5, 0.75, 43.5) (14.5, 0.75, 46.5) on bodies 1
extrude "Extrude56" add 2 faces at (7.1667, 0, 44.5) (1.1667, 0, 23.5) along direction (0, 1, 0) blind 1.5 on bodies 1 bodies 1
extrude "Extrude57" cut 1 faces at (10.6667, -0.5, 37.878) along direction (0, 1, 0) blind 0.5 on bodies 1 bodies 1
sketch "Sketch17" plane through (0, 1.5, 0) normal (0, 1, 0) x (-1, 0, 0)
  circle A0 centre (11.5, 6) radius 1.25
  circle A1 centre (-11.5, 6) radius 1.25
  circle A2 centre (11.5, 64) radius 1.25
  circle A3 centre (-11.5, 64) radius 1.25
  circle A4 centre (-13, 60) radius 1.25
  circle A5 centre (-12.5, 12) radius 1.25
  circle A6 centre (4.5, 12) radius 1.25
  circle A7 centre (5, 60) radius 1.25
  line L0 (8, 61.5) -> (14, 61.5)
  line L1 (14, 61.5) -> (14, 70)
  line L2 (14, 70) -> (11, 70)
  line L3 (11, 70) -> (11, 72)
  line L4 (11, 72) -> (-19, 72)
  line L5 (-19, 72) -> (-19, 70)
  line L6 (-19, 70) -> (-22, 70)
  line L7 (-22, 70) -> (-22, 65)
  line L8 (-22, 65) -> (-16, 65)
  line L9 (-16, 65) -> (-16, 41)
  line L10 (-16, 41) -> (-15, 41)
  line L11 (-15, 41) -> (-15, 29)
  line L12 (-15, 29) -> (-16, 29)
  line L13 (-16, 29) -> (-16, 5)
  line L14 (-16, 5) -> (-22, 5)
  line L15 (-22, 5) -> (-22, 0)
  line L16 (-22, 0) -> (-19, 0)
  line L17 (-19, 0) -> (-19, -2)
  line L18 (-19, -2) -> (11, -2)
  line L19 (11, -2) -> (11, 0)
  line L20 (11, 0) -> (14, 0)
  line L21 (14, 0) -> (14, 8.5)
  line L22 (14, 8.5) -> (8, 8.5)
  line L23 (8, 8.5) -> (8, 61.5)
  line L24 (3.75, 60) -> (3.75, 64)
  line L25 (3.25, 6) -> (3.25, 12)
  line L26 (-10.25, 64) -> (-8.25, 64)
  line L27 (3.75, 60) -> (1.75, 60)
  line L28 (3.25, 12) -> (1.25, 12)
  line L29 (-10.25, 6) -> (-8.25, 6)
  line L30 (1.75, 60) -> (1.75, 12)
  line L31 (-8.25, 6) -> (-8.25, 64)
  line L32 (-8.25, 6) -> (-8.25, 4)
  line L33 (-8.25, 64) -> (-8.25, 66)
  line L34 (-8.25, 66) -> (-8.25, 67)
  line L35 (-8.25, 72) -> (-8.25, 69)
  line L36 (1.75, 60) -> (1.75, 61.5)
  line L37 (1.75, 72) -> (1.75, 69)
  line L38 (-8.25, -2) -> (-8.25, 1)
  line L39 (1.75, 12) -> (1.75, 10)
  line L40 (1.75, -2) -> (1.75, 1)
  line L41 (-10.25, 64) -> (-8.25, 64)
  line L42 (-10.25, 6) -> (-8.25, 6)
  line L43 (1.75, 12) -> (1.75, 14)
  line L44 (-8.25, 14) -> (-8.25, 10)
  line L45 (1.75, 10) -> (1.75, 14)
  line L46 (1.75, 60) -> (1.75, 58)
  line L47 (-8.25, 58) -> (-8.25, 61.5)
  line L48 (1.75, 61.5) -> (1.75, 58)
  line L49 (-8.25, 4) -> (-8.25, 4)
  line L50 (-8.25, 66) -> (-8.25, 69)
  line L51 (-5.25, 69) -> (-5.25, 69)
  line L52 (1.75, 10) -> (1.75, 4)
  line L53 (-5.25, 1) -> (-1.25, 1)
  arc A8 (-1.25, 1) -> (1.75, 4) centre (-1.25, 4) ccw
  arc A9 (-8.25, 4) -> (-5.25, 1) centre (-5.25, 4) ccw
  line L54 (1.75, 10.5) -> (1.75, 11)
  line L55 (1.75, 10) -> (1.75, 10.5)
  line L56 (1.75, 10.5) -> (-8.25, 10.5)
  line L57 (-8.25, 10.5) -> (-8.25, 13.5)
  line L58 (-8.25, 13.5) -> (1.75, 13.5)
  line L59 (1.75, 13.5) -> (1.75, 10.5)
  line L60 (1.75, 58) -> (1.75, 58.5)
  line L61 (1.75, 58.5) -> (-8.25, 58.5)
  line L62 (-8.25, 58.5) -> (-8.25, 61.5)
  line L63 (-8.25, 61.5) -> (1.75, 61.5)
  line L64 (1.75, 61.5) -> (1.75, 58.5)
  arc A10 (-5.25, 69) -> (-8.25, 66) centre (-5.25, 66) ccw
  line L65 (-1.25, 69) -> (-5.25, 69)
  line L66 (1.75, 61.5) -> (1.75, 66)
  arc A11 (1.75, 66) -> (-1.25, 69) centre (-1.25, 66) ccw
  dimension "d230" = 13.5
  dimension "d231" = 2
  dimension "d232" = 2
  dimension "d233" = 2
  dimension "d234" = 2
  dimension "d235" = 3
  dimension "d236" = 3
  dimension "d243" = 4
  dimension "d245" = 3
  dimension "d246" = 3
  dimension "d247" = 3
  dimension "d248" = 0.5
  dimension "d249" = 3
  dimension "d250" = 3
  dimension "d251" = 3
  constraint coincident A3 L26.start
  constraint parallel L6 L41
  constraint coincident A7 L24.start
  constraint coincident L24.end L41
  constraint tangent A7 L24
  constraint perpendicular L24 L41
  constraint coincident A1 L29.start
  constraint perpendicular L23 L42
  constraint coincident A6 L25.end
  constraint tangent A6 L25
  constraint perpendicular L25 L42
  constraint perpendicular L7 L26
  constraint perpendicular L24 L27
  constraint perpendicular L25 L28
  constraint perpendicular L13 L29
  constraint vertical L30
  constraint coincident L28 L30.end
  constraint perpendicular L31 L41
  constraint coincident L18 L38.start
  constraint perpendicular L18 L32
  constraint coincident L4 L35.start
  constraint perpendicular L4 L33
  constraint coincident L33 L34.end
  constraint perpendicular L4 L35
  constraint coincident L4 L37.start
  constraint perpendicular L4 L36
  constraint coincident L36 L37.end
  constraint perpendicular L4 L37
  constraint perpendicular L18 L38
  constraint coincident L18 L40.start
  constraint perpendicular L18 L39
  constraint coincident L39 L40.end
  constraint coincident L35.start L33
  constraint coincident L38.start L32
  constraint coincident L40.start L39
  constraint coincident L30 L43.end
  constraint perpendicular L28 L43
  constraint vertical L44
  constraint vertical L45
  constraint coincident L30 L46.end
  constraint perpendicular L27 L46
  constraint vertical L47
  constraint vertical L48
  constraint coincident L40.end L53
  constraint coincident L40.end L52
  constraint tangent L53 A8
  constraint tangent L52 A8
  constraint coincident L38.end L49
  constraint coincident L38.end L53
  constraint tangent L53 A9
  constraint midpoint L39 L54.end
  constraint horizontal L56
  constraint vertical L57
  constraint horizontal L58
  constraint vertical L59
  constraint horizontal L61
  constraint vertical L62
  constraint horizontal L63
  constraint vertical L64
  constraint coincident L35.start L34
  constraint coincident L35.end L51
  constraint tangent L34 A10
  constraint tangent A10 L65
  constraint parallel L37 L66
  constraint coincident L37.end L65
  constraint tangent L66 A11
  constraint tangent L65 A11
  measures "d230" distance of L29.start L25.start
  measures "d231" distance of L26.start L26.end
  measures "d232" distance of L24.start L27.end
  measures "d233" distance of L25.end L28.end
  measures "d234" distance of L29.start L29.end
  measures "d235" distance of L35.start L35.end
  measures "d236" distance of L38.start L38.end
  measures "d243" distance of L43.end L39.end
  measures "d245" radius of A8
  measures "d246" radius of A9
  measures "d247" distance of L54.start L58.end
  measures "d248" distance of L46.end L60.end
  measures "d249" distance of L60.end L36.end
  measures "d250" radius of A10
  measures "d251" radius of A11
extrude "Extrude59" cut sketch "Sketch17" against normal blind 100 contours L30 L31 L43 L44 L45 L46 L47 L48 L58 L60 L61 | L31 L33 L63 A10 L65 L66 A11 | L31 L32 L39 L44 L45 L52 L53 A8 A9 L55 L56 bodies 1
extrude "Extrude58" cut sketch "Sketch17" against normal blind 10 contours L30 L31 L39 L43 L44 L45 L54 L56 L57 L58 L59 bodies 1
extrude "Extrude60" add sketch "Sketch17" against normal blind 3 contours L30 L31 L39 L43 L44 L45 L54 L56 L57 L58 L59 bodies 1
fillet "Fillet13" radius 3 4 edges at (8.25, 0, 10.5) (-1.75, 0, 10.5) (8.25, 0, 13.5) (-1.75, 0, 13.5) on bodies 1
fillet "Fillet14" radius 3 4 edges at (8.25, 0, 58.5) (-1.75, 0, 58.5) (8.25, 0, 61.5) (-1.75, 0, 61.5) on bodies 1
fillet "Fillet16" radius 3 4 edges at (-8, 0, 8.5) (-8, 0, 61.5) (-14, 0, 61.5) (-14, 0, 8.5) on bodies 1
fillet "Fillet18" radius 3 1 edges at (15, 1.5, 35) on bodies 1
fillet "Fillet19" radius 1.5 1 edges at (15, -1.5, 35) on bodies 1
fillet "Fillet20" radius 3 1 edges at (14, 1.5, 41) on bodies 1
fillet "Fillet21" radius 3 1 edges at (14, 1.5, 29) on bodies 1
sketch "Sketch18" plane through (0, -9, 0) normal (0, -1, 0) x (1, 0, 0)
  line L0 (15, 41) -> (15, 29)
  line L1 (15, 29) -> (16, 29)
  line L2 (16, 29) -> (16, 41)
  line L3 (16, 41) -> (15, 41)
  line L4 (15, 29) -> (14, 29)
  line L5 (14, 29) -> (14, 41)
  line L6 (14, 41) -> (15, 41)
  line L7 (15, 41) -> (15, 29)
  constraint horizontal L4
  constraint vertical L5
  constraint horizontal L6
  constraint vertical L7
  constraint coincident L0.end L1.start
extrude "Extrude61" cut sketch "Sketch18" against normal blind 7.5 contours L0 L4 L5 L6 L7 bodies 1
fillet "Fillet22" radius 3 2 edges at (15.5, -1.5, 29) (15.5, -1.5, 41) on bodies 1
fillet "Fillet23" radius 1 1 edges at (15, -1.5, 35) on bodies 1
fillet "Fillet24" radius 3 8 edges at (-12.5, -1.5, 0) (20.5, -1.5, 0) (20.5, -1.5, 70) (-12.5, -1.5, 70) (-12.5, 1.5, 70) (20.5, 1.5, 70) (20.5, 1.5, 0) (-12.5, 1.5, 0) on bodies 1
fillet "Fillet25" radius 3 8 edges at (-11, 1.5, 0.5) (19, 1.5, 0.5) (-11, -1.5, 0.5) (19, -1.5, 0.5) (19, -1.5, 69.5) (-11, -1.5, 69.5) (19, 1.5, 69.5) (-11, 1.5, 69.5) on bodies 1
sketch "Sketch19" plane through (0, 1.5, 0) normal (0, 1, 0) x (-1, 0, 0)
  line L0 (8, 67) -> (8, 72)
  line L1 (8, 72) -> (-16, 72)
  line L2 (-16, 72) -> (-16, 67)
  line L3 (-16, 67) -> (-22, 67)
  line L4 (-22, 67) -> (-22, 65)
  line L5 (-22, 65) -> (-16, 65)
  line L6 (-16, 65) -> (-16, 44)
  line L7 (-16, 44) -> (-12, 44)
  line L8 (-12, 44) -> (-12, 26)
  line L9 (-12, 26) -> (-16, 26)
  line L10 (-16, 5) -> (-22, 5)
  line L11 (-22, 5) -> (-22, 3)
  line L12 (-22, 3) -> (-16, 3)
  line L13 (-16, 3) -> (-16, -2)
  line L14 (-16, -2) -> (8, -2)
  line L15 (8, -2) -> (8, 3)
  line L16 (8, 3) -> (14, 3)
  line L17 (14, 3) -> (14, 5.5)
  arc A0 (14, 5.5) -> (11, 8.5) centre (11, 5.5) ccw
  arc A1 (8, 11.5) -> (11, 8.5) centre (11, 11.5) ccw
  line L18 (8, 11.5) -> (8, 58.5)
  arc A2 (11, 61.5) -> (8, 58.5) centre (11, 58.5) ccw
  arc A3 (11, 61.5) -> (14, 64.5) centre (11, 64.5) ccw
  line L19 (14, 64.5) -> (14, 67)
  line L20 (14, 67) -> (8, 67)
  line L21 (1.75, 66) -> (1.75, 64.5)
  arc A4 (-1.25, 61.5) -> (1.75, 64.5) centre (-1.25, 64.5) ccw
  line L22 (-1.25, 61.5) -> (-5.25, 61.5)
  arc A5 (-8.25, 64.5) -> (-5.25, 61.5) centre (-5.25, 64.5) ccw
  line L23 (-8.25, 64.5) -> (-8.25, 66)
  arc A6 (-5.25, 69) -> (-8.25, 66) centre (-5.25, 66) ccw
  line L24 (-5.25, 69) -> (-1.25, 69)
  arc A7 (1.75, 66) -> (-1.25, 69) centre (-1.25, 66) ccw
  line L25 (1.75, 7.5) -> (1.75, 4)
  arc A8 (-1.25, 1) -> (1.75, 4) centre (-1.25, 4) ccw
  line L26 (-1.25, 1) -> (-5.25, 1)
  arc A9 (-8.25, 4) -> (-5.25, 1) centre (-5.25, 4) ccw
  line L27 (-8.25, 4) -> (-8.25, 7.5)
  arc A10 (-5.25, 10.5) -> (-8.25, 7.5) centre (-5.25, 7.5) ccw
  line L28 (-5.25, 10.5) -> (-1.25, 10.5)
  arc A11 (1.75, 7.5) -> (-1.25, 10.5) centre (-1.25, 7.5) ccw
  circle A12 centre (11.5, 6) radius 1.25
  circle A13 centre (-11.5, 6) radius 1.25
  circle A14 centre (11.5, 64) radius 1.25
  circle A15 centre (-11.5, 64) radius 1.25
  circle A16 centre (-13, 60) radius 1.25
  circle A17 centre (-12.5, 12) radius 1.25
  circle A18 centre (4.5, 12) radius 1.25
  circle A19 centre (5, 60) radius 1.25
  line L29 (-8.25, 16.5) -> (-8.25, 55.5)
  arc A20 (-5.25, 58.5) -> (-8.25, 55.5) centre (-5.25, 55.5) ccw
  line L30 (-5.25, 58.5) -> (-1.25, 58.5)
  arc A21 (1.75, 55.5) -> (-1.25, 58.5) centre (-1.25, 55.5) ccw
  line L31 (1.75, 55.5) -> (1.75, 16.5)
  arc A22 (-1.25, 13.5) -> (1.75, 16.5) centre (-1.25, 16.5) ccw
  line L32 (-1.25, 13.5) -> (-5.25, 13.5)
  arc A23 (-8.25, 16.5) -> (-5.25, 13.5) centre (-5.25, 16.5) ccw
  circle A24 centre (5, 60) radius 1.75
  circle A25 centre (-13, 60) radius 1.75
  circle A26 centre (4.5, 12) radius 1.75
  circle A27 centre (-12.5, 12) radius 1.75
  line L33 (4.5, 12) -> (5.75, 12)
  line L34 (-12.5, 12) -> (-14.25, 12)
  line L35 (-12.5, 8.75) -> (4.5, 8.75)
  line L36 (4.5, 8.75) -> (7.75, 8.75)
  line L37 (7.75, 8.75) -> (7.75, 22.75)
  line L38 (-12.5, 8.75) -> (-15.75, 8.75)
  line L39 (-15.75, 8.75) -> (-15.75, 22.75)
  line L40 (-15.75, 22.75) -> (7.75, 22.75)
  line L41 (-12.5, 12) -> (-12.5, 10.25)
  line L42 (4.5, 10.75) -> (4.5, 10.25)
  line L43 (-13, 60) -> (-16.25, 60)
  line L44 (5, 60) -> (5, 63.25)
  line L45 (5, 60) -> (6.75, 60)
  line L46 (-16.25, 60) -> (-16.25, 63.25)
  line L47 (-16.25, 63.25) -> (8.25, 63.25)
  line L48 (8.25, 63.25) -> (8.25, 46.25)
  line L49 (-16.25, 63.25) -> (-16.25, 46.25)
  line L50 (-16.25, 46.25) -> (8.25, 46.25)
  line L51 (-16, 26) -> (-16, 5)
  dimension "d284" = 3.5
  dimension "d285" = 3.5
  dimension "d292" = 3.5
  dimension "d293" = 3.5
  dimension "d302" = 3.25
  dimension "d304" = 3.25
  dimension "d305" = 3.25
  dimension "d306" = 14
  dimension "d307" = 3.25
  dimension "d308" = 14
  dimension "d309" = 3.25
  dimension "d311" = 3.25
  dimension "d313" = 3.25
  dimension "d314" = 24.5
  dimension "d315" = 17
  dimension "d316" = 17
  constraint concentric A19 A24
  constraint concentric A16 A25
  constraint concentric A18 A26
  constraint concentric A17 A27
  constraint coincident A18.centre A26.centre
  constraint coincident A17.centre A27.centre
  constraint perpendicular L33 L42
  constraint perpendicular L35 L42
  constraint perpendicular L36 L42
  constraint perpendicular L36 L37
  constraint perpendicular L38 L39
  constraint coincident A27 L34.end
  constraint coincident A27 L41.end
  constraint coincident A26 L42.end
  constraint coincident A18 L42.start
  constraint coincident A18 L33.end
  constraint coincident A16.centre A25.centre
  constraint perpendicular L6 L43
  constraint coincident A19.centre A24.centre
  constraint vertical L44
  constraint perpendicular L44 L45
  constraint vertical L46
  constraint perpendicular L46 L47
  constraint perpendicular L47 L48
  constraint perpendicular L47 L49
  constraint coincident A24 L45.end
  measures "d284" diameter of A24
  measures "d285" diameter of A25
  measures "d292" diameter of A26
  measures "d293" diameter of A27
  measures "d302" distance of A17.centre L35.start
  measures "d304" distance of A18.centre L35.end
  measures "d305" distance of L35.end L36.end
  measures "d306" distance of L36.end L37.end
  measures "d307" distance of L35.start L38.end
  measures "d308" distance of L38.end L39.end
  measures "d309" distance of A16.centre L43.end
  measures "d311" distance of A19.centre L44.end
  measures "d313" distance of L43.end L46.end
  measures "d314" distance of L46.end L47.end
  measures "d315" distance of L47.end L48.end
  measures "d316" distance of L46.end L49.end
extrude "Extrude62" add sketch "Sketch19" along normal blind 1.6 separate body contours L18 A2 L48 L50 | L6 L18 A2 A4 L22 A5 A15 L29 A20 L30 A21 L31 L47 L48 L50 | L6 L43 L46 L47 L49 | L6 L43 L49 L50 makes body 3
extrude "Extrude63" add sketch "Sketch19" along normal blind 1.6 separate body contours A10 L28 A11 L29 L31 A22 L32 A23 L35 L36 L37 L38 L39 L40 makes body 4
move_face "OffsetFaces1" offset -0.5 5 faces at (2.5833, 2.0333, 13.5) (-1.6958, 2.5667, 15.9322) (-1.75, 2.0333, 20.6667) (7.8481, 2.5667, 15) (8.25, 2.0333, 18.5833) on bodies 4
extrude "Extrude64" cut 2 faces at (13.4167, 2.0333, 22.75) (-4.0833, 2.0333, 22.75) along direction (0, 0, -1) blind 0.5 on bodies 4 bodies 4
extrude "Extrude65" cut 1 faces at (-7.75, 2.0333, 13.25) along direction (1, 0, 0) blind 0.5 on bodies 4 bodies 4
extrude "Extrude66" cut 1 faces at (15.75, 2.5667, 17.75) along direction (-1, 0, 0) blind 0.5 on bodies 4 bodies 4
extrude "Extrude67" cut 2 faces at (12.8257, 2.0333, 8.75) (-3.4015, 2.0333, 8.75) along direction (0, 0, 1) blind 0.5 on bodies 4 bodies 4
move_face "OffsetFaces2" offset -0.5 3 faces at (0.9652, 2.0333, 10.4864) (3.9167, 2.5667, 10.5) (5.5348, 2.5667, 10.4864) on bodies 4
fillet "Fillet26" radius 2 8 edges at (8.75, 2.3, 22.25) (15.25, 2.3, 22.25) (15.25, 2.3, 9.25) (8.2811, 2.3, 9.25) (-1.7811, 2.3, 9.25) (-7.25, 2.3, 9.25) (-7.25, 2.3, 22.25) (-2.25, 2.3, 22.25) on bodies 4
extrude "Extrude68" add sketch "Sketch19" along normal blind 1.6 contours A15 L47 picked at (-11.5885, 63.0928) bodies 3
move_face "OffsetFaces3" offset -0.5 3 faces at (6.365, 2.5667, 58.2851) (3.9167, 2.0333, 58.5) (-1.3481, 2.5667, 57) on bodies 3
extrude "Extrude69" cut 2 faces at (13.75, 2.0333, 46.25) (-6.25, 2.5667, 46.25) along direction (0, 0, 1) blind 0.5 on bodies 3 bodies 3
extrude "Extrude70" cut 1 faces at (16.25, 2.0333, 52.25) along direction (-1, 0, 0) blind 0.5 on bodies 3 bodies 3
extrude "Extrude71" cut 1 faces at (-8.25, 2.0333, 57.75) along direction (1, 0, 0) blind 0.5 on bodies 3 bodies 3
extrude "Extrude72" cut 2 faces at (13.1591, 2.0333, 63.25) (-5.6591, 2.5667, 63.25) along direction (0, 0, -1) blind 0.5 on bodies 3 bodies 3
move_face "OffsetFaces5" offset -0.5 3 faces at (7.3182, 2.5667, 62.3269) (2.5833, 2.0333, 61.5) (0.9652, 2.5667, 61.5136) on bodies 3
fillet "Fillet27" radius 2 8 edges at (15.75, 2.3, 62.75) (8.2811, 2.3, 62.75) (-1.7811, 2.3, 62.75) (-7.75, 2.3, 62.75) (-7.75, 2.3, 46.75) (-2.25, 2.3, 46.75) (8.75, 2.3, 46.75) (15.75, 2.3, 46.75) on bodies 3
extrude "Extrude73" cut 1 faces at (11.0833, 3.1, 51) along direction (0, -1, 0) blind 0.1 on bodies 3 bodies 3
extrude "Extrude74" cut 1 faces at (12.1231, 3.1, 16.8317) along direction (0, -1, 0) blind 0.5 on bodies 4 bodies 4
extrude "Extrude75" add 1 faces at (12.1231, 2.6, 16.8317) along direction (0, 1, 0) blind 0.4 on bodies 4 bodies 4
extrude "Extrude76" cut 1 faces at (15.3333, 9, 33) along direction (0, -1, 0) blind 1 on bodies 1 bodies 1
extrude "Extrude77" cut 1 faces at (15.3333, -9, 37) along direction (0, 1, 0) blind 1 on bodies 1 bodies 1